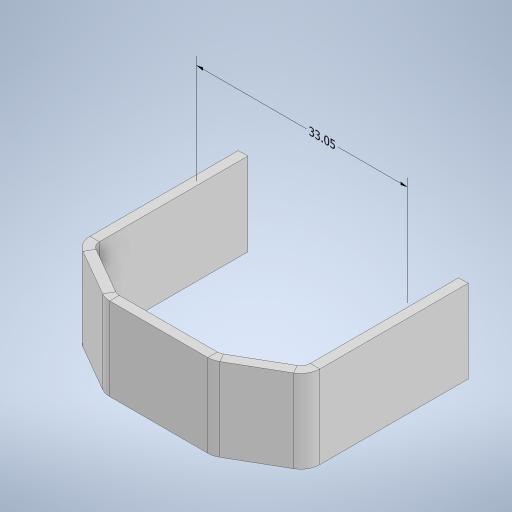
# Autodesk Inventor part: Head_cover_CNC
Saved by Autodesk Inventor 2024.1 (Build 281209000, 209)
## iProperties
Created: 2024-02-18
Part Number: Head_cover_CNC
Material: 一般
Document SubType Name: Sheet Metal
Designer: hibik
Density: 1 g/cm^3
Sheet Metal Rule: Robomech
Appearance: 既定
Author: hibik
Autodesk Inventor part; units mm, degrees
ref_plane "YZ Plane" through (0, 0, 0) normal (1, 0, 0) x (0, 1, 0)
ref_plane "XZ Plane" through (0, 0, 0) normal (0, 1, 0) x (-1, 0, 0)
ref_plane "XY Plane" through (0, 0, 0) normal (0, 0, 1) x (1, 0, 0)
sketch "スケッチ1" plane through (0, 0, 0) normal (0, 0, 1) x (1, 0, 0)
  line L0 (6.5, 6.5) -> (-6.5, 6.5)
  line L1 (-6.5, 6.5) -> (-6.5, -6.5)
  line L2 (-6.5, -6.5) -> (6.5, -6.5)
  line L3 (6.5, -6.5) -> (6.5, 6.5)
  line L4 (6.5, 6.5) -> (-6.5, -6.5) construction
  line L5 (-6.5, 6.5) -> (6.5, -6.5) construction
  line L6 (6.5, -6.5) -> (-6.5, -6.5)
  line L7 (6.5, 6.5) -> (-6.5, 6.5)
  line L8 (-6.5, 6.5) -> (-8.5, 6.5)
  line L9 (-8.5, 6.5) -> (-8.5, -6.5)
  line L10 (-8.5, -6.5) -> (-6.5, -6.5)
  line L11 (-6.5, -6.5) -> (-6.5, 6.5)
  line L12 (6.5, 6.5) -> (8.5, 6.5)
  line L13 (8.5, 6.5) -> (8.5, -6.5)
  line L14 (8.5, -6.5) -> (6.5, -6.5)
  line L15 (6.5, -6.5) -> (6.5, 6.5)
  point P0 (0, 0)
  dimension "d0" = 13
  dimension "d1" = 13
  dimension "d4" = 2
  measures "d0" distance of L2.end L1.end
  measures "d1" distance of L1.end L0.end
  measures "d4" distance of L7.end L8.end
extrude "プレート1" add sketch "スケッチ1" along normal blind 1.5
sketch "スケッチ2" plane through (7.75, -6.5, 0.201) normal (0.5, 0, 0.8660254) x (0, 1, 0)
  line L0 (13, 0) -> (0, 0)
  line L1 (0, 0) -> (0, -11)
  line L2 (0, -11) -> (13, -11)
  line L3 (13, -11) -> (13, 0)
  constraints: 6 end point, 1 horizontal, 1 perpendicular, 1 vertical
edge flange "フランジ1" height 11 angle 30 thickness 1.5 bend radius 1.5 thickness toward (0.5, 0, 0.8660254) relief straight relief width 1.5 relief depth 0.75 corner gap 1.5 corner form 0 edges at (8.5, 0, 0) (-8.5, 0, 0) wall of the first edge with corners at (7.75, 6.5, 0.201) (7.75, -6.5, 0.201) (17.2763, -6.5, -5.299) (17.2763, 6.5, -5.299)
bend "曲げ1"
corner "コーナー1"
sketch "スケッチ3" plane through (-16.5263, 6.5, -4) normal (-1, 0, 0) x (0, -1, 0)
  line L0 (13, 0) -> (0, 0)
  line L1 (0, 0) -> (0, -25)
  line L2 (0, -25) -> (13, -25)
  line L3 (13, -25) -> (13, 0)
  constraints: 6 end point, 1 horizontal, 1 perpendicular, 1 vertical
edge flange "フランジ2" height 25 angle 60 thickness 1.5 bend radius 1.5 thickness toward (-1, 0, 0) relief straight relief width 1.5 relief depth 0.75 corner gap 1.5 corner form 0 edges at (-17.2763, 0, -5.299) (17.2763, 0, -5.299) wall of the first edge with corners at (-16.5263, -6.5, -4) (-16.5263, 6.5, -4) (-16.5263, 6.5, -29) (-16.5263, -6.5, -29)
bend "曲げ2"
corner "コーナー2"
equation "\"d2\" = Thickness"
equation "\"d5\" = BendReliefWidth"
equation "\"d6\" = BendReliefDepth"
equation "\"d7\" = MinimumRemnant"
equation "\"d8\" = TransitionRadius"
equation "\"d11\" = BendRadius"
equation "\"d12\" = CornerReliefSize"
equation "\"d13\" = GapSize"
equation "\"d14\" = JacobiRadiusSize"
equation "\"d15\" = BendReliefWidth"
equation "\"d16\" = BendReliefDepth"
equation "\"d17\" = MinimumRemnant"
equation "\"d18\" = TransitionRadius"
equation "\"d21\" = BendRadius"
equation "\"d22\" = CornerReliefSize"
equation "\"d23\" = GapSize"
equation "\"d24\" = JacobiRadiusSize"
equation "\"BendRadius\" = Thickness"
equation "\"BendReliefWidth\" = Thickness"
equation "\"BendReliefDepth\" = 0.5 * Thickness"
equation "\"CornerReliefSize\" = 4 * Thickness"
equation "\"MinimumRemnant\" = 2 * Thickness"
equation "\"TransitionRadius\" = BendRadius"
equation "\"JacobiRadiusSize\" = BendRadius"
equation "\"GapSize\" = Thickness"
equation "\"Thickness\" = 1.5"
